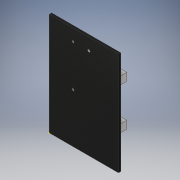
# Autodesk Inventor part: back plate
Saved by Autodesk Inventor 2019 (Build 230136000, 136)
## iProperties
Created: 2020-02-19
Part Number: back plate
Material: Generic
Document SubType Name: Modeling
Designer: LENOVO
Density: 1 g/cm^3
Appearance: Default
Author: LENOVO
Autodesk Inventor part; units mm, degrees
ref_plane "YZ Plane" through (0, 0, 0) normal (1, 0, 0) x (0, 1, 0)
ref_plane "XZ Plane" through (0, 0, 0) normal (0, 1, 0) x (-1, 0, 0)
ref_plane "XY Plane" through (0, 0, 0) normal (0, 0, 1) x (1, 0, 0)
sketch "Sketch1" plane through (0, 0, 0) normal (0, 0, 1) x (1, 0, 0)
  line L0 (0, 0) -> (350, 0)
  line L1 (350, 0) -> (350, 520)
  line L2 (350, 520) -> (0, 520)
  line L3 (0, 520) -> (0, 0)
  dimension "d0" = 350
  dimension "d1" = 520
  constraints: 8 end point, 2 parallel, 1 horizontal, 1 perpendicular
  measures "d0" distance of L2.end L1.end
  measures "d1" distance of L1.end L0.end
extrude "Extrusion1" add sketch "Sketch1" along normal blind 12
sketch "Sketch2" plane through (0, 0, 12) normal (0, 0, 1) x (1, 0, 0)
  line L0 (0, 120) -> (350, 120)
  line L1 (350, 120) -> (350, 370)
  line L2 (350, 0) -> (350, 520) projected
  line L3 (350, 370) -> (0, 370)
  line L4 (0, 520) -> (0, 0) projected
  line L5 (0, 370) -> (0, 520)
  line L6 (350, 520) -> (0, 520) projected
  line L7 (0, 520) -> (350, 520)
  line L8 (350, 520) -> (350, 370)
  circle A0 centre (120, 460) radius 6.5
  circle A1 centre (120, 250) radius 6.5
  dimension "d6" = 13
  dimension "d7" = 13
  constraints: 12 end point, 2 centre point, 2 collinear, 2 perpendicular, 2 point on line, 1 horizontal
  measures "d6" diameter of A0
  measures "d7" diameter of A1
extrude "Extrusion2" cut sketch "Sketch2" against normal blind 12 contours A0 | A1
thread "Thread1" size "M14x2" class "6H" standard "ANSI Metric M Profile" full length
thread "Thread2" size "M14x2" class "6H" standard "ANSI Metric M Profile" full length
sketch "Sketch3" plane through (0, 0, 0) normal (0, 0, -1) x (-1, 0, 0)
  circle A0 centre (-200, 460) radius 6.5
  point P0 (0, 0)
  dimension "d14" = 13
  constraints: 1 centre point
  measures "d14" diameter of A0
extrude "Extrusion3" cut sketch "Sketch3" against normal blind 120
sketch "Sketch4" plane through (0, 0, 12) normal (0, 0, 1) x (1, 0, 0)
  point P0 (0, 0)
sketch "Sketch5" plane through (0, 0, 0) normal (0, 0, -1) x (-1, 0, 0)
  point P0 (0, 0)
sketch "Sketch6" plane through (0, 0, 0) normal (0, 0, -1) x (-1, 0, 0)
  line L0 (-330, 400) -> (-250, 400)
  line L1 (-250, 400) -> (-250, 360)
  line L2 (-250, 360) -> (-330, 360)
  line L3 (-330, 360) -> (-330, 400)
  line L4 (-330, 190) -> (-250, 190)
  line L5 (-250, 190) -> (-250, 150)
  line L6 (-250, 150) -> (-330, 150)
  line L7 (-330, 150) -> (-330, 190)
  point P0 (0, 0)
  dimension "d17" = 80
  dimension "d18" = 40
  dimension "d19" = 80
  dimension "d20" = 40
  constraints: 16 end point, 4 parallel, 2 horizontal, 2 perpendicular, 1 point on line
  measures "d17" distance of L1.end L2.end
  measures "d18" distance of L0.end L1.end
  measures "d19" distance of L5.end L6.end
  measures "d20" distance of L4.end L5.end
extrude "Extrusion4" add sketch "Sketch6" along normal blind 50
body "Solid1"
